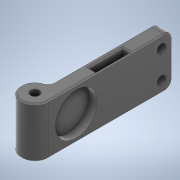
# Autodesk Inventor part: 08-04-01-003_clutchPaddleLever
Saved by Autodesk Inventor 2020 (Build 240168000, 168)
## iProperties
Created: 2021-07-31
Part Number: 08-04-01-003_clutchPaddleLever
Material: ABS-Kunststoff(1)
Document SubType Name: Modeling
Designer: Eric
Density: 1.06 g/cm^3
Appearance: Glatt - Weiß(1)
Author: Eric
## iProperties of the stored document _3D-Druck.ipt
Created: 2021-08-28
Part Number: _3D-Druck
Material: Generisch
Document SubType Name: Modeling
Designer: Eric
Density: 1 g/cm^3
Appearance: Vorgabe
Author: Eric
Autodesk Inventor part; units mm, degrees
ref_plane "YZ Plane" through (0, 0, 0) normal (1, 0, 0) x (0, 1, 0)
ref_plane "XZ Plane" through (0, 0, 0) normal (0, 1, 0) x (-1, 0, 0)
ref_plane "XY Plane" through (0, 0, 0) normal (0, 0, 1) x (1, 0, 0)
sketch "Skizze1" plane through (0, 0, 0) normal (0, 1, 0) x (-1, 0, 0)
  circle A0 centre (0, 0) radius 1.6
  arc A1 (1.4286, -4.7916) -> (-5, 0) centre (0, 0) ccw
  arc A2 (1.4286, -4.7916) -> (0, -6.7082) centre (2, -6.7082) ccw
  line L0 (0, -6.7082) -> (0, -45)
  line L1 (0, -45) -> (-5, -45)
  line L2 (-5, -45) -> (-5, 0)
  dimension "d0" = 3.2
  dimension "d2" = 3.4
  dimension "d3" = 2
  dimension "d4" = 45
  constraints: 6 end point, 4 point on circle, 3 centre point, 3 tangent, 1 coincident, 1 concentric, 1 parallel, 1 perpendicular, 1 vertical, 1 vertical alignment
  measures "d0" diameter of A0
  measures "d2" radial gap between concentric circles of A1 A0
  measures "d3" radius of A2
  measures "d4" distance of L1.end L2.end
extrude "Extrusion1" add sketch "Skizze1" along normal blind 18.2
fillet "Rundung1" radius 3 2 edges at (2.5, 18.2, -45) (2.5, 0, -45)
chamfer "Fase1" distance 0.5 angle 45 14 edges at (0, 18.2, -24.3541) (-0.3964, 18.2, -5.513) (-2.9881, 18.2, 4.0089) (5, 18.2, -21) (5, 17.3213, -44.1213) (5, 9.1, -45) (5, 0.8787, -44.1213) (5, 0, -21) (-2.9881, 0, 4.0089) (-0.3964, 0, -5.513) (0, 0, -24.3541) (0, 0.8787, -44.1213) (0, 9.1, -45) (0, 17.3213, -44.1213)
sketch "Skizze2" plane through (0, 0.5, -6.7082) normal (-1, 0, 0) x (0, 0, 1)
  circle A0 centre (-34.2918, 3.6) radius 1.6
  circle A1 centre (-34.2918, 13.6) radius 1.6
  line L0 (-34.2918, 13.6) -> (-34.2918, 3.6) construction
  line L1 (-37.7918, 2.5) -> (-37.7918, 14.7) construction
  line L2 (-38.2918, 14.7) -> (-38.2918, 2.5) projected
  point P0 (6.7082, -0.5)
  point P1 (-34.2918, 8.6)
  point P2 (-37.7918, 8.6)
  dimension "d11" = 10
  dimension "d12" = 3.2
  dimension "d13" = 4
  constraints: 2 centre point, 2 end point, 2 midpoint, 1 equal radius, 1 horizontal alignment, 1 vertical
  measures "d11" distance of L0.start L0.end
  measures "d12" diameter of A0
  measures "d13" distance between parallel lines of L2 L0
extrude "Extrusion2" cut sketch "Skizze2" against normal blind 19
sketch "Skizze3" plane through (5, 0.5, 0) normal (1, 0, 0) x (0, 0, -1)
  line L0 (-5, 0) -> (-5, 17.2) projected
  circle A0 centre (10, 8.6) radius 7.6
  circle A1 centre (24, 8.6) radius 6.1
  point P0 (0, -0.5)
  point P1 (-5, 8.6)
  dimension "d16" = 15
  dimension "d17" = 15.2
  dimension "d23" = 29
  dimension "d24" = 12.2
  constraints: 2 centre point, 2 horizontal alignment, 1 midpoint
  measures "d16" distance from line of A0.centre L0
  measures "d17" diameter of A0
  measures "d23" distance from line of A1.centre L0
  measures "d24" diameter of A1
extrude "Extrusion3" cut sketch "Skizze3" against normal blind 3 contours A0
sketch "Skizze7" plane through (0, 18.2, 0) normal (0, 1, 0) x (1, 0, 0)
  line L0 (1.8, 17.9) -> (4.6, 17.9)
  line L1 (4.6, 17.9) -> (4.6, 30.1)
  line L2 (4.6, 30.1) -> (1.8, 30.1)
  line L3 (1.8, 30.1) -> (1.8, 17.9)
  arc A0 (-1.4286, 4.7916) -> (5, 0) centre (0, 0) ccw projected
  line L4 (5, 0) -> (5, 42) projected
  dimension "d27" = 5
  dimension "d28" = 12.2
  dimension "d29" = 2.8
  dimension "d30" = 0.4
  dimension "d33" = 17.9
  constraints: 8 end point, 2 parallel, 1 horizontal, 1 perpendicular
  measures "d27" radius of A0
  measures "d28" distance of L2.end L0.start
  measures "d29" distance of L0.start L0.end
  measures "d30" distance between parallel lines of L4 L1
  measures "d33" distance from line of L0 point (0, 0)
extrude "Extrusion5" cut sketch "Skizze7" against normal blind 15.2
fillet "Rundung2" radius 6.1 2 edges at (3.2, 3, -17.9) (3.2, 3, -30.1)
chamfer "Fase2" distance 0.5 angle 45 3 edges at (3.15, 18.2, -17.9) (3.15, 18.2, -30.1) (1.8, 18.2, -24)
